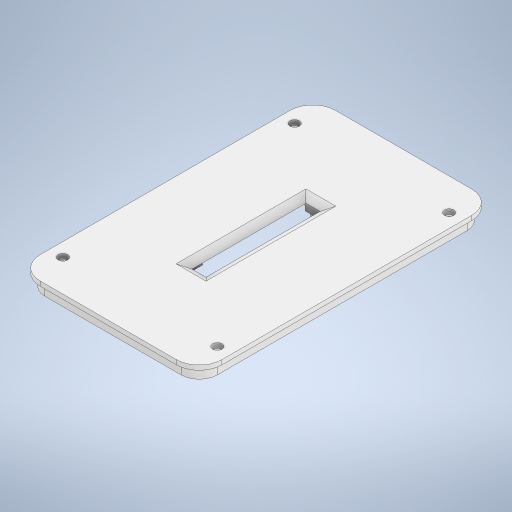
# Autodesk Inventor part: TOP
Saved by Autodesk Inventor 2023 (Build 270158000, 158)
## iProperties
Created: 2023-03-14
Part Number: TOP
Material: Generic
Document SubType Name: Modeling
Designer: Amos Yu
Density: 1 g/cm^3
Appearance: White
Author: Amos Yu
Autodesk Inventor part; units mm, degrees
ref_plane "YZ Plane" through (0, 0, 0) normal (1, 0, 0) x (0, 1, 0)
ref_plane "XZ Plane" through (0, 0, 0) normal (0, 1, 0) x (-1, 0, 0)
ref_plane "XY Plane" through (0, 0, 0) normal (0, 0, 1) x (1, 0, 0)
sketch "Sketch1" plane through (0, 0, 0) normal (0, 1, 0) x (-1, 0, 0)
  line L0 (-10, 0) -> (-70, 0)
  line L1 (-80, -10) -> (-80, -120)
  line L2 (-70, -130) -> (-10, -130)
  line L3 (0, -120) -> (0, -10)
  arc A0 (0, -10) -> (-10, 0) centre (-10, -10) ccw
  arc A1 (-70, 0) -> (-80, -10) centre (-70, -10) ccw
  arc A2 (-80, -120) -> (-70, -130) centre (-70, -120) ccw
  arc A3 (-10, -130) -> (0, -120) centre (-10, -120) ccw
  point P0 (0, 0)
  point P1 (-80, -130)
  point P2 (-80, 0)
  point P3 (0, -130)
  dimension "d0" = 80
  dimension "d1" = 130
  dimension "d2" = 10
  constraints: 8 end point, 8 point on circle, 8 point on line, 8 tangent, 4 centre point, 3 equal radius, 2 parallel, 1 horizontal, 1 perpendicular
  measures "d0" distance of point (0, -130) point (-80, -130)
  measures "d1" distance of point (-80, -130) point (-80, 0)
  measures "d2" radius of A0
extrude "Extrusion1" add sketch "Sketch1" against normal blind 2
sketch "Sketch2" plane through (0, -2, 0) normal (0, -1, 0) x (1, 0, 0)
  line L0 (80, -120) -> (80, -10) projected
  line L1 (70, 0) -> (10, 0) projected
  line L2 (0, -10) -> (0, -120) projected
  line L3 (10, -130) -> (70, -130) projected
  line L4 (70, -2.1) -> (10, -2.1)
  line L5 (2.1, -10) -> (2.1, -120)
  line L6 (10, -127.9) -> (70, -127.9)
  line L7 (77.9, -120) -> (77.9, -10)
  arc A0 (77.9, -10) -> (70, -2.1) centre (70, -10) ccw
  arc A1 (10, -2.1) -> (2.1, -10) centre (10, -10) ccw
  arc A2 (2.1, -120) -> (10, -127.9) centre (10, -120) ccw
  arc A3 (70, -127.9) -> (77.9, -120) centre (70, -120) ccw
  line L8 (70, -4.1) -> (10, -4.1)
  arc A4 (10, -4.1) -> (4.1, -10) centre (10, -10) ccw
  line L9 (4.1, -10) -> (4.1, -120)
  arc A5 (4.1, -120) -> (10, -125.9) centre (10, -120) ccw
  line L10 (10, -125.9) -> (70, -125.9)
  arc A6 (70, -125.9) -> (75.9, -120) centre (70, -120) ccw
  line L11 (75.9, -120) -> (75.9, -10)
  arc A7 (75.9, -10) -> (70, -4.1) centre (70, -10) ccw
  point P0 (0, 0)
  dimension "d5" = 2.1
  dimension "d6" = 2.1
  dimension "d7" = 2.1
  dimension "d8" = 2.1
  dimension "d9" = 7.9
  dimension "d10" = 2
  constraints: 16 end point, 16 point on circle, 8 centre point, 8 tangent, 4 parallel, 3 equal radius, 2 perpendicular, 1 horizontal, 7 other
  measures "d5" distance between parallel lines of L3 L6
  measures "d6" distance between parallel lines of L0 L7
  measures "d7" distance between parallel lines of L1 L4
  measures "d8" distance between parallel lines of L2 L5
  measures "d9" radius of A0
  measures "d10" radial gap between concentric circles of A0 A7
extrude "Extrusion2" add sketch "Sketch2" along normal blind 4.9
sketch "Sketch3" plane through (0, -2, 0) normal (0, -1, 0) x (1, 0, 0)
  circle A0 centre (6, -14) radius 1.1
  circle A1 centre (6, -14) radius 3.1
  line L0 (70, 0) -> (10, 0) projected
  line L1 (0, -10) -> (0, -120) projected
  circle A2 centre (74, -14) radius 1.1
  circle A3 centre (74, -14) radius 3.1
  circle A4 centre (6, -116) radius 1.1
  circle A5 centre (6, -116) radius 3.1
  circle A6 centre (74, -116) radius 1.1
  circle A7 centre (74, -116) radius 3.1
  point P0 (0, 0)
  dimension "d13" = 2.2
  dimension "d14" = 2
  dimension "d15" = 14
  dimension "d16" = 6
  dimension "d19" = 68
  dimension "d22" = 102
  constraints: 8 centre point, 4 coincident, 1 horizontal, 1 vertical, 12 other
  measures "d13" diameter of A0
  measures "d14" radial gap between concentric circles of A1 A0
  measures "d15" distance from line of L0 A0.centre
  measures "d16" distance from line of L1 A0.centre
  measures "d19" distance of A0.centre A2.centre
  measures "d22" distance of A0.centre A4.centre
extrude "Extrusion3" add sketch "Sketch3" along normal up to surface (4.9 mm away)
extrude "Extrusion4" cut sketch "Sketch3" along normal up to surface (4.9 mm away) contours A0 | A2 | A4 | A6
sketch "Sketch4" plane through (0, 0, 0) normal (0, 1, 0) x (1, 0, 0)
  circle A0 centre (6, 14) radius 2.1
  line L0 (0, 120) -> (0, 10) projected
  line L1 (10, 0) -> (70, 0) projected
  circle A1 centre (6, 116) radius 2.1
  circle A2 centre (74, 14) radius 2.1
  circle A3 centre (74, 116) radius 2.1
  point P0 (0, 0)
  dimension "d29" = 4.2
  dimension "d30" = 14
  dimension "d31" = 6
  dimension "d34" = 102
  dimension "d37" = 68
  constraints: 4 centre point, 1 horizontal, 1 vertical, 6 other
  measures "d29" diameter of A0
  measures "d30" vertical distance of point (0, 0) A0.centre
  measures "d31" horizontal distance of point (0, 0) A0.centre
  measures "d34" distance of A0.centre A1.centre
  measures "d37" distance of A0.centre A2.centre
extrude "Extrusion5" cut sketch "Sketch4" against normal blind 2.1
ref_plane "Work Plane1" through (10, 0, -100) normal (0, 0, 1) x (1, 0, 0)
sketch "Sketch6" plane through (10, 0, -100) normal (0, 0, 1) x (1, 0, 0)
  line L0 (19, -2) -> (41, -2)
  line L1 (41, -2) -> (41, -16)
  line L2 (41, -16) -> (19, -16)
  line L3 (19, -16) -> (19, -2)
  line L4 (19, -2) -> (41, -16) construction
  line L5 (41, -2) -> (19, -16) construction
  line L6 (60, 0) -> (0, 0) projected
  circle A0 centre (22.3, -6) radius 1.1
  circle A1 centre (37.7, -6) radius 1.1
  line L7 (22.3, -6) -> (37.7, -6) construction
  point P0 (-10, 0)
  point P1 (30, -9)
  point P2 (30, 0)
  point P3 (30, -2)
  point P4 (30, -6)
  dimension "d46" = 22
  dimension "d47" = 14
  dimension "d48" = 2
  dimension "d49" = 2.2
  dimension "d50" = 2.2
  dimension "d54" = 15.4
  dimension "d55" = 10
  constraints: 14 end point, 5 midpoint, 2 centre point, 2 horizontal, 2 parallel, 2 vertical alignment, 1 horizontal alignment, 1 perpendicular
  measures "d46" distance of L1.end L2.end
  measures "d47" distance of L0.end L1.end
  measures "d48" distance between parallel lines of L6 L0
  measures "d49" diameter of A0
  measures "d50" diameter of A1
  measures "d54" distance of L7.end L7.start
  measures "d55" distance from line of L2 point (30, -6)
extrude "Extrusion6" add sketch "Sketch6" against normal blind 2
fillet "Fillet1" radius 2 3 edges at (51, -2, -101) (40, -2, -102) (29, -2, -101)
sketch "Sketch7" plane through (0, -2, 0) normal (0, -1, 0) x (1, 0, 0)
  line L0 (43.1, -39.9) -> (36.9, -39.9)
  line L1 (36.9, -39.9) -> (36.9, -90.1)
  line L2 (36.9, -90.1) -> (43.1, -90.1)
  line L3 (43.1, -90.1) -> (43.1, -39.9)
  line L4 (10, 0) -> (70, 0) projected
  line L5 (0, -120) -> (0, -10) projected
  point P0 (0, 0)
  point P1 (40, -39.9)
  point P2 (40, 0)
  point P3 (36.9, -65)
  point P4 (0, -65)
  dimension "d61" = 50.2
  dimension "d62" = 6.2
  constraints: 8 end point, 4 midpoint, 2 parallel, 1 horizontal, 1 horizontal alignment, 1 perpendicular, 1 vertical alignment
  measures "d61" distance of L0.end L1.end
  measures "d62" distance of L0.start L0.end
extrude "Extrusion7" cut sketch "Sketch7" against normal up to surface (2 mm away) draft 60
ref_plane "Work Plane2" through (40, -2, -120) normal (-1, 0, 0) x (0, 0, 1)
sketch "Sketch8" plane through (0, -2, 0) normal (0, -1, 0) x (1, 0, 0)
  line L0 (43.8, -37.5) -> (41.8, -37.5)
  line L1 (41.8, -37.5) -> (41.8, -39.5)
  line L2 (41.8, -39.5) -> (43.8, -39.5)
  line L3 (43.8, -39.5) -> (43.8, -37.5)
  line L4 (80, -120) -> (80, -10) projected
  line L5 (43.8, -90.5) -> (36.2, -90.5)
  line L6 (36.2, -90.5) -> (36.2, -92.5)
  line L7 (36.2, -92.5) -> (43.8, -92.5)
  line L8 (43.8, -92.5) -> (43.8, -90.5)
  line L9 (43.1, -90.1) -> (36.9, -90.1) construction
  point P0 (0, 0)
  point P1 (40, -90.1)
  point P2 (40, -90.5)
  dimension "d63" = 39.5
  dimension "d64" = 2
  dimension "d65" = 2
  dimension "d69" = 38.2
  dimension "d83" = 51
  dimension "d84" = 2
  constraints: 16 end point, 4 parallel, 2 horizontal, 2 midpoint, 2 perpendicular, 2 vertical alignment
  measures "d63" vertical distance of L1.end point (0, 0)
  measures "d64" distance of L1.end L2.end
  measures "d65" distance of L2.end L0.start
  measures "d69" distance from line of L4 L0.end
  measures "d83" distance between parallel lines of L2 L5
  measures "d84" distance of L5.end L6.end
extrude "Extrusion8" add sketch "Sketch8" along normal blind 5.7 contours L3 L2 L1 L0
extrude "Extrusion10" add sketch "Sketch8" along normal blind 3.5 contours L8 L7 L6 L5
sketch "Sketch9" plane through (43.8, -2, -39.5) normal (0, 0, -1) x (-1, 0, 0)
  line L0 (33.8, 0) -> (-26.2, 0) construction
  line L1 (-7.3, 0) -> (-1.6, -5.7)
  line L2 (-1.6, -5.7) -> (-9.3, -5.7)
  line L3 (-9.3, -5.7) -> (-9.3, 0)
  line L4 (-7.3, 0) -> (-9.3, 0)
  line L5 (19.5, -5.7) -> (19.5, 0)
  line L6 (17.5, 0) -> (11.8, -5.7)
  line L7 (11.8, -5.7) -> (19.5, -5.7)
  line L8 (17.5, 0) -> (19.5, 0)
  point P0 (43.8, 2)
  dimension "d70" = 51.1
  dimension "d71" = 45
  dimension "d72" = 45
  dimension "d73" = 5.7
  dimension "d74" = 24.8
  dimension "d75" = 2
  dimension "d76" = 2
  constraints: 16 end point, 4 perpendicular, 4 point on line, 1 collinear, 1 horizontal alignment, 1 parallel
  measures "d70" horizontal distance of point (43.8, 2) L1.start
  measures "d71" angle of L0 L1
  measures "d72" angle of L6 L0
  measures "d73" distance of L5.start L5.end
  measures "d74" distance of L1.start L6.start
  measures "d75" distance of L3.end L1.start
  measures "d76" distance of L5.end L6.start
extrude "Extrusion9" add sketch "Sketch9" along normal blind 12
fillet "Fillet2" radius 2 9 edges at (24.3, -2, -45.5) (53.1, -2, -45.5) (25.3, -2, -39.5) (42.8, -2, -37.5) (52.1, -2, -39.5) (43.8, -2, -38.5) (36.2, -2, -91.5) (40, -2, -92.5) (43.8, -2, -91.5)
chamfer "Chamfer1" distance 2 angle 45 2 edges at (48.25, -4.85, -51.5) (29.15, -4.85, -51.5)
equation "\"d0\" = total_width"
equation "\"d1\" = total_depth"
equation "\"d2\" = fillet_outer_radius"
equation "\"d3\" = thickness"
equation "\"d5\" = thickness + tol"
equation "\"d6\" = thickness + tol"
equation "\"d7\" = thickness + tol"
equation "\"d8\" = thickness + tol"
equation "\"d9\" = -thickness + fillet_outer_radius - tol"
equation "\"d10\" = thickness"
equation "\"d11\" = lip_height - tol"
equation "\"d13\" = bolt_thread_diameter + 2 * tol"
equation "\"d14\" = thickness"
equation "\"d15\" = bolt_inset_depth"
equation "\"d16\" = bolt_inset_width"
equation "\"d19\" = total_width - 2 * bolt_inset_width"
equation "\"d22\" = total_depth - 2 * bolt_inset_depth"
equation "\"d25\" = lip_height - tol"
equation "\"d29\" = bolt_head_diameter + 2 * tol"
equation "\"d30\" = bolt_inset_depth"
equation "\"d31\" = bolt_inset_width"
equation "\"d34\" = total_depth - 2 * bolt_inset_depth"
equation "\"d37\" = total_width - 2 * bolt_inset_width"
equation "\"d40\" = bolt_head_height + tol"
equation "\"d46\" = adxl_mount_width"
equation "\"d47\" = adxl_mount_height"
equation "\"d48\" = thickness"
equation "\"d49\" = bolt_thread_diameter + 2 * tol"
equation "\"d50\" = d51 + 2 * d52"
equation "\"d54\" = adxl_hole_separation_width"
equation "\"d56\" = thickness"
equation "\"d58\" = thickness"
equation "\"d61\" = led_hole_depth + 2 * tol"
equation "\"d62\" = led_hole_width + 2 * tol"
equation "\"d83\" = led_depth + 2 * tol"
equation "\"d84\" = thickness"
equation "\"d67\" = led_height + thickness + 4 * tol"
equation "\"d85\" = led_height + 2 * tol"
equation "\"d73\" = led_height + thickness + 4 * tol"
equation "\"d74\" = led_housing_width + 8 * tol"
equation "\"d75\" = thickness"
equation "\"d76\" = thickness"
equation "\"d77\" = led_housing_rail_depth"
equation "\"d79\" = thickness"
equation "\"d80\" = thickness"
equation "\"adxl_mount_width\" = 22"
equation "\"led_hole_width\" = 6"
equation "\"led_depth\" = 50.8"
equation "\"fillet_outer_radius\" = 10"
equation "\"thickness\" = 2"
equation "\"tol\" = 0.1"
equation "\"lip_height\" = 5"
equation "\"bolt_thread_diameter\" = 2"
equation "\"bolt_inset_depth\" = 14"
equation "\"bolt_inset_width\" = 6"
equation "\"total_width\" = 80"
equation "\"total_depth\" = 130"
equation "\"bolt_head_diameter\" = 4"
equation "\"bolt_head_height\" = 2"
equation "\"adxl_mount_height\" = 14"
equation "\"d51\" = 2"
equation "\"d52\" = 0.1"
equation "\"adxl_hole_separation_width\" = 15.4"
equation "\"led_hole_depth\" = 50"
equation "\"led_height\" = 3.3"
equation "\"led_housing_width\" = 24"
equation "\"led_housing_rail_depth\" = 12"
body "Solid1"
